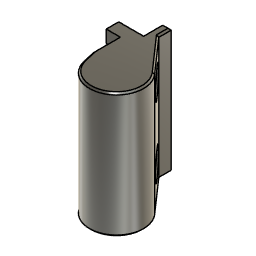
mini_fridge_top_latch_left (Autodesk Fusion 360 design; units mm, degrees)
Autodesk Fusion 360 part; units mm, degrees
sketch "Sketch1" plane through (0, 0, 0) normal (0, 0, 1) x (1, 0, 0)
  line L0 (-2.35, 12.52) -> (-7, 12.52)
  line L1 (-7, 12.52) -> (-7, 10.52)
  line L2 (-7, 10.52) -> (-11.5, 10.52)
  line L3 (-11.5, 10.52) -> (-11.5, 7.52)
  line L4 (-11.5, 7.52) -> (-7, 7.52)
  line L5 (-7, 7.52) -> (-7, 1.5)
  line L6 (-2.35, 12.52) -> (4.882336, 4.291014)
  line L7 (-7, 1.5) -> (-6.341463, -1.426829)
  arc A0 (-6.341463, -1.426829) -> (4.882336, 4.291014) centre (0, 0) ccw
  dimension "d1" = 13
  dimension "d2" = 7
  dimension "d3" = 12.52
  dimension "d4" = 4.65
  dimension "d5" = 2
  dimension "d6" = 4.5
  dimension "d7" = 3
  dimension "d8" = 6.02
  constraint coincident A0.centre origin
  constraint horizontal L0
  constraint perpendicular L0 L1
  constraint perpendicular L1 L2
  constraint perpendicular L2 L3
  constraint perpendicular L3 L4
  constraint perpendicular L4 L5
  constraint tangent L6 A0
  constraint tangent L7 A0
  measures "d1" diameter of A0
  measures "d2" horizontal distance of A0.centre L0.end
  measures "d3" vertical distance of A0.centre L0.end
  measures "d4" distance of L0.start L0.end
  measures "d5" distance of L0.end L1.end
  measures "d6" distance of L1.end L2.end
  measures "d7" distance of L2.end L3.end
  measures "d8" distance of L4.end L5.end
extrude "Extrude1" add sketch "Sketch1" along normal blind 30
sketch "Sketch2" plane through (-11.5, 0, 0) normal (-1, 0, 0) x (0, -1, 0)
  line L0 (-10.52, 0) -> (-7.52, 0)
  line L1 (-7.52, 0) -> (-7.52, 30)
  line L2 (-7.52, 30) -> (-10.52, 30)
  line L3 (-10.52, 30) -> (-10.52, 0)
  circle A0 centre (-9.02, 6.5) radius 2.75
  circle A1 centre (-9.02, 23.5) radius 2.75
  dimension "d11" = 5.5
  dimension "d12" = 5.5
  dimension "d13" = 6.5
  dimension "d14" = 6.5
  measures "d11" diameter of A0
  measures "d12" diameter of A1
  measures "d13" distance of L0 A0.centre
  measures "d14" distance of L2 A1.centre
extrude "Extrude2" cut sketch "Sketch2" against normal blind 27 contours L3 A0 | L1 L3 A0 | L1 A0 | L3 A1 | L1 L3 A1 | L1 A1 picked at (-10.958448, 6.199736) picked at (-9.52, 5.731705) picked at (-7.140043, 6.243186) picked at (-10.715223, 22.902553) picked at (-9.52, 22.731705) picked at (-6.841134, 23.335551)
sketch "Sketch3" plane through (-11.5, 0, 0) normal (-1, 0, 0) x (0, -1, 0)
  arc A0 (-7.52, 8.804886) -> (-10.52, 8.804886) centre (-9.02, 6.5) ccw
  line L0 (-7.52, 8.804886) -> (-7.52, 21.195114)
  arc A1 (-10.52, 21.195114) -> (-7.52, 21.195114) centre (-9.02, 23.5) ccw
  line L1 (-10.52, 21.195114) -> (-10.52, 8.804886)
  circle A2 centre (-9.02, 23.5) radius 1.7
  circle A3 centre (-9.02, 6.5) radius 1.7
  circle A4 centre (-9.02, 23.5) radius 2.75
  circle A5 centre (-9.02, 6.5) radius 2.75
  dimension "d17" = 3.4
  dimension "d18" = 3.4
  dimension "d19" = 5.5
  dimension "d20" = 5.5
  constraint concentric A1 A2
  constraint concentric A0 A3
  constraint concentric A1 A4
  constraint concentric A3 A5
  measures "d17" diameter of A2
  measures "d18" diameter of A3
  measures "d19" diameter of A4
  measures "d20" diameter of A5
extrude "Extrude3" add sketch "Sketch3" against normal blind 8.9 contours A0 A5 | A1 A4 picked at (-10.480929, 8.397685) picked at (-10.480929, 21.602315)
sketch "Sketch4" plane through (0, 0, 0) normal (0, 0, -1) x (1, 0, 0)
  line L0 (-7, -12.52) -> (-2.35, -12.52)
  line L1 (-2.35, -12.52) -> (4.882336, -4.291014)
  arc A0 (4.882336, -4.291014) -> (-6.341463, 1.426829) centre (0, 0) ccw
  line L2 (-6.341463, 1.426829) -> (-7, -1.5)
  line L3 (-7, -1.5) -> (-7, -7.52)
  line L4 (-7, -7.52) -> (-11.5, -7.52)
  line L5 (-11.5, -7.52) -> (-11.5, -10.52)
  line L6 (-11.5, -10.52) -> (-7, -10.52)
  line L7 (-7, -10.52) -> (-7, -12.52)
  line L8 (-7, -12.52) -> (-11.5, -12.52)
  line L9 (-11.5, -12.52) -> (-11.5, -10.52)
  line L10 (-11.5, -10.52) -> (-7, -10.52)
  line L11 (-7, -10.52) -> (-7, -12.52)
  line L12 (-7, -7.52) -> (-11.5, -7.52)
  line L13 (-11.5, -7.52) -> (-11.5, -5.132341)
  line L14 (-11.5, -5.132341) -> (-7, -5.132341)
  line L15 (-7, -5.132341) -> (-7, -7.52)
  constraint horizontal L8
  constraint vertical L9
  constraint horizontal L10
  constraint vertical L11
  constraint coincident L5.end L6.start
  constraint coincident L0.start L7.end
  constraint horizontal L12
  constraint vertical L13
  constraint horizontal L14
  constraint vertical L15
  constraint coincident L3.end L4.start
extrude "Extrude4" cut sketch "Sketch4" against normal blind 37 contours L6 L7 L8 L9 L10 L11 | L3 L4 L12 L13 L14 L15 picked at (-8.5, -11.853333) picked at (-8.5, -6.724114)
sketch "Sketch5" plane through (0, 12.52, 0) normal (0, 1, 0) x (-1, 0, 0)
  line L0 (2.35, 0) -> (7, 0)
  line L1 (7, 0) -> (7, 30)
  line L2 (7, 30) -> (2.35, 30)
  line L3 (2.35, 30) -> (2.35, 0)
  line L4 (7, 27) -> (13.720787, 27)
  line L5 (13.720787, 27) -> (13.720787, 20)
  line L6 (13.720787, 20) -> (7, 20)
  line L7 (7, 20) -> (7, 27)
  line L8 (7, 10) -> (13.720787, 10)
  line L9 (13.720787, 10) -> (13.720787, 3)
  line L10 (13.720787, 3) -> (7, 3)
  line L11 (7, 3) -> (7, 10)
  line L12 (7, 30) -> (11.5, 30)
  line L13 (7, 0) -> (11.5, 0)
  dimension "d25" = 3
  dimension "d26" = 7
  dimension "d27" = 3
  dimension "d28" = 7
  constraint horizontal L4
  constraint vertical L5
  constraint horizontal L6
  constraint vertical L7
  constraint coincident L1 L4.start
  constraint horizontal L8
  constraint vertical L9
  constraint horizontal L10
  constraint vertical L11
  constraint coincident L1 L8.start
  measures "d25" distance of L4 L12
  measures "d27" distance of L10 L13
extrude "Extrude5" cut sketch "Sketch5" against normal blind 27 contours L1 L8 L9 L10 L11 | L1 L4 L5 L6 L7 picked at (11.480525, 5.333333) picked at (9.240262, 22.333333)
sketch "Sketch7" plane through (0, 10.52, 0) normal (0, 1, 0) x (-1, 0, 0)
  line L0 (11.5, 20) -> (7, 20)
  line L1 (7, 20) -> (7, 10)
  line L2 (7, 10) -> (11.5, 10)
  line L3 (11.5, 10) -> (11.5, 20)
  line L4 (10, 32.726892) -> (15.810138, 32.726892)
  line L5 (15.810138, 32.726892) -> (15.810138, -2.648108)
  line L6 (15.810138, -2.648108) -> (10, -2.648108)
  line L7 (10, -2.648108) -> (10, 32.726892)
  line L8 (7, 0) -> (7, 30)
  dimension "d31" = 3
  constraint horizontal L4
  constraint vertical L5
  constraint horizontal L6
  constraint vertical L7
  measures "d31" distance of L7 L8
extrude "Extrude6" cut sketch "Sketch7" against normal blind 17 contours L0 L2 L3 L7 | L0 L2 L3 L4 L5 L6 L7 picked at (10.5, 16.666667) picked at (12.436713, 28.484595)
sketch "Sketch8" plane through (-10, 0, 0) normal (-1, 0, 0) x (0, -1, 0)
  line L0 (-7.52, 20) -> (-10.52, 20)
  line L1 (-10.52, 20) -> (-10.52, 10)
  line L2 (-10.52, 10) -> (-7.52, 10)
  line L3 (-7.52, 10) -> (-7.52, 20)
  line L4 (-18.312737, 20.75) -> (-10.52, 20.75)
  line L5 (-10.52, 20.75) -> (-10.52, -5.80303)
  line L6 (-10.52, -5.80303) -> (-18.312737, -5.80303)
  line L7 (-18.312737, -5.80303) -> (-18.312737, 20.75)
  line L8 (-7.52, 0) -> (-1.5, 0)
  line L9 (-12.52, 0) -> (-12.52, 30)
  dimension "d34" = 20.75
  dimension "d35" = 2
  constraint horizontal L4
  constraint vertical L5
  constraint horizontal L6
  constraint vertical L7
  measures "d34" distance of L4 L8
  measures "d35" distance of L5 L9
extrude "Extrude7" cut sketch "Sketch8" against normal blind 6 contours L1 L4 L5 L6 L7 picked at (-15.715158, 8.315657)
extrude "Extrude8" add 1 faces at (-4.45, 12.52, 26.916667) along direction (0, 1, 0) blind 1
extrude "Extrude9" add 1 faces at (-4.45, 13.52, 26.916667) along direction (0, 1, 0) blind 1
chamfer "Chamfer1" distance 2 distance2 2 1 edges at (-4.675, 14.52, 30) measured on face at (-4.45, 14.52, 26.916667)
extrude "Extrude10" add 1 faces at (-4.45, 14.52, 25.583333) along direction (0, 1, 0) blind 1
delete_face "DeleteFace1" 2 faces at (-3.9, 15.186667, 28) (-3.9, 13.853333, 28.666667)
chamfer "Chamfer2" distance 3 distance2 3 1 edges at (-4.675, 15.52, 30) measured on face at (-4.45, 15.52, 26.916667)
sketch "Sketch9" plane through (0, 0, 0) normal (0, 0, -1) x (1, 0, 0)
  line L0 (-4, -10.52) -> (-4, -15.52)
  line L1 (-4, -15.52) -> (-2.35, -15.52)
  line L2 (-2.35, -15.52) -> (-2.35, -12.52)
  line L3 (-2.35, -12.52) -> (4.882336, -4.291014)
  arc A0 (4.882336, -4.291014) -> (-6.341463, 1.426829) centre (0, 0) ccw
  line L4 (-6.341463, 1.426829) -> (-7, -1.5)
  line L5 (-7, -1.5) -> (-7, -7.52)
  line L6 (-7, -7.52) -> (-10, -7.52)
  line L7 (-10, -7.52) -> (-10, -10.52)
  line L8 (-10, -10.52) -> (-4, -10.52)
  circle A1 centre (0, 0) radius 2.6
  dimension "d48" = 5.2
  constraint concentric A0 A1
  measures "d48" diameter of A1
extrude "Extrude11" cut sketch "Sketch9" against normal blind 26 contours A1 picked at (0.90431, -0.249748)
sketch "Sketch10" plane through (0, 0, 0) normal (0, 0, -1) x (1, 0, 0)
  circle A0 centre (0, 0) radius 2.6
  line L0 (-4, -10.52) -> (-4, -15.52)
  line L1 (-4, -15.52) -> (-2.35, -15.52)
  line L2 (-2.35, -15.52) -> (-2.35, -12.52)
  line L3 (-2.35, -12.52) -> (4.882336, -4.291014)
  arc A1 (4.882336, -4.291014) -> (-6.341463, 1.426829) centre (0, 0) ccw
  line L4 (-6.341463, 1.426829) -> (-7, -1.5)
  line L5 (-7, -1.5) -> (-7, -7.52)
  line L6 (-7, -7.52) -> (-10, -7.52)
  line L7 (-10, -7.52) -> (-10, -10.52)
  line L8 (-10, -10.52) -> (-4, -10.52)
  circle A2 centre (0, 0) radius 3.5
  dimension "d51" = 7
  constraint concentric A0 A2
  measures "d51" diameter of A2
extrude "Extrude12" cut sketch "Sketch10" against normal blind 17 contours A2 picked at (3.177289, -0.303053)
chamfer "Chamfer3" distance 1 distance2 1 1 edges at (-3.263146, -1.265654, 0) measured on face at (1.10372, 6.741087, 0)
chamfer "Chamfer4" distance 0.4 distance2 0.4 7 edges at (2.950541, -5.791745, 0) (1.266168, 8.405507, 0) (-6.670732, 0.036585, 0) (-7, 4.51, 0) (-2.35, 14.02, 0) (-3.175, 15.52, 0) (-4, 13.02, 0) measured on face at (5.084833, 4.049009, 20) measured on face at (-4.416667, 7.312371, 0) measured on face at (-6.560976, -0.45122, 10) measured on face at (-7, 3.506667, 13.333333) measured on face at (-2.35, 13.52, 19) measured on face at (-4.45, 15.52, 24.916667) measured on face at (-4.416667, 7.312371, 0)
chamfer "Chamfer5" distance 0.4 distance2 0.4 5 edges at (1.266168, 8.405507, 30) (-6.670732, 0.036585, 30) (2.950541, -5.791745, 30) (-7, 4.51, 30) (-7, 11.52, 30) measured on face at (-1.489221, 8.110338, 30) measured on face at (-1.489221, 8.110338, 30) measured on face at (-1.489221, 8.110338, 30) measured on face at (-1.489221, 8.110338, 30) measured on face at (-7, 3.506667, 13.466667)
chamfer "Chamfer6" distance 0.4 distance2 0.4 1 edges at (-2.35, 12.217041, 30) measured on face at (-2.35, 13.52, 19)
chamfer "Chamfer7" distance 0.4 distance2 0.4 2 edges at (-1.690836, 11.77, 23.5) (-1.690836, 11.77, 6.5) measured on face at (1.133213, 8.556783, 28.481768) measured on face at (1.133213, 8.556783, 28.481768)
extrude "Extrude13" cut 1 faces at (-5, 13.853333, 20.75) along direction (0, 0, 1) blind 32
delete_face "DeleteFace2" 1 faces at (-3.45, 13.653307, 28.866693)
chamfer "Chamfer8" distance 0.4 distance2 0.4 1 edges at (-3.375, 15.52, 30) measured on face at (1.486948, 0.297923, 30)
